Autodesk Fusion 360 part; units mm, degrees
(part 4 of 7)
  spline S44 degree 5 poles (-7.921, 8.6736) (-7.9244, 8.6773) (-7.9314, 8.6848) (-7.9421, 8.6957) (-7.957, 8.7098) (-7.9762, 8.7266) (-7.9959, 8.743) (-8.016, 8.759) (-8.0362, 8.7749) (-8.0566, 8.7907) (-8.077, 8.8063) (-8.0977, 8.8219) (-8.1185, 8.8372) (-8.1396, 8.8522) (-8.1609, 8.867) (-8.1824, 8.8816) (-8.2042, 8.896) (-8.226, 8.9102) (-8.2481, 8.9242) (-8.2702, 8.9382) (-8.2925, 8.9519) (-8.3149, 8.9656) (-8.3375, 8.9791) (-8.3602, 8.9924) (-8.3831, 9.0056) (-8.4061, 9.0186) (-8.4292, 9.0314) (-8.4524, 9.0442) (-8.4758, 9.0568) (-8.4993, 9.0692) (-8.5229, 9.0816) (-8.5466, 9.0938) (-8.5704, 9.1058) (-8.5943, 9.1178) (-8.6184, 9.1296) (-8.6426, 9.1413) (-8.6668, 9.1528) (-8.6912, 9.1642) (-8.7157, 9.1755) (-8.7402, 9.1867) (-8.7649, 9.1978) (-8.7897, 9.2087) (-8.8146, 9.2195) (-8.8395, 9.2302) (-8.8646, 9.2408) (-8.8897, 9.2512) (-8.915, 9.2616) (-8.9403, 9.2718) (-8.9658, 9.2819) (-8.9913, 9.2919) (-9.0169, 9.3018) (-9.0426, 9.3115) (-9.0684, 9.3212) (-9.0942, 9.3307) (-9.1202, 9.3401) (-9.1462, 9.3494) (-9.1723, 9.3586) (-9.1985, 9.3677) (-9.2248, 9.3767) (-9.2512, 9.3856) (-9.2776, 9.3943) (-9.3041, 9.403) (-9.3307, 9.4115) (-9.3574, 9.4199) (-9.3841, 9.4282) (-9.4109, 9.4364) (-9.4378, 9.4445) (-9.4648, 9.4525) (-9.4918, 9.4604) (-9.5189, 9.4682) (-9.5461, 9.4758) (-9.5679, 9.4819) (-9.5843, 9.4864) (-9.5953, 9.4894) (-9.6007, 9.4908) knots 0 0 0 0 0 0 0.01428571 0.02857143 0.04285714 0.05714286 0.07142857 0.08571429 0.1 0.11428571 0.12857143 0.14285714 0.15714286 0.17142857 0.18571429 0.2 0.21428571 0.22857143 0.24285714 0.25714286 0.27142857 0.28571429 0.3 0.31428571 0.32857143 0.34285714 0.35714286 0.37142857 0.38571429 0.4 0.41428571 0.42857143 0.44285714 0.45714286 0.47142857 0.48571429 0.5 0.51428571 0.52857143 0.54285714 0.55714286 0.57142857 0.58571429 0.6 0.61428571 0.62857143 0.64285714 0.65714286 0.67142857 0.68571429 0.7 0.71428571 0.72857143 0.74285714 0.75714286 0.77142857 0.78571429 0.8 0.81428571 0.82857143 0.84285714 0.85714286 0.87142857 0.88571429 0.9 0.91428571 0.92857143 0.94285714 0.95714286 0.97142857 0.98571429 1 1 1 1 1 1
  arc A90 (-9.6007, 9.4908) -> (-10.0749, 8.9858) centre (0, 0) ccw
  spline S45 degree 5 poles (-10.0749, 8.9858) (-10.0731, 8.9805) (-10.0695, 8.9698) (-10.064, 8.9537) (-10.0566, 8.9323) (-10.0472, 8.9057) (-10.0377, 8.8791) (-10.0282, 8.8526) (-10.0185, 8.8262) (-10.0087, 8.7998) (-9.9989, 8.7736) (-9.9889, 8.7474) (-9.9788, 8.7213) (-9.9686, 8.6953) (-9.9583, 8.6694) (-9.9479, 8.6436) (-9.9374, 8.6178) (-9.9268, 8.5922) (-9.9161, 8.5666) (-9.9053, 8.5411) (-9.8944, 8.5157) (-9.8833, 8.4904) (-9.8722, 8.4652) (-9.8609, 8.4401) (-9.8496, 8.415) (-9.8381, 8.3901) (-9.8266, 8.3653) (-9.8149, 8.3405) (-9.8031, 8.3159) (-9.7912, 8.2913) (-9.7792, 8.2669) (-9.767, 8.2425) (-9.7548, 8.2183) (-9.7424, 8.1941) (-9.73, 8.1701) (-9.7174, 8.1462) (-9.7047, 8.1223) (-9.6919, 8.0986) (-9.6789, 8.075) (-9.6659, 8.0515) (-9.6527, 8.0281) (-9.6394, 8.0049) (-9.626, 7.9817) (-9.6125, 7.9587) (-9.5988, 7.9358) (-9.585, 7.913) (-9.5711, 7.8904) (-9.5571, 7.8679) (-9.5429, 7.8455) (-9.5286, 7.8232) (-9.5142, 7.8011) (-9.4996, 7.7791) (-9.4849, 7.7572) (-9.47, 7.7356) (-9.455, 7.7141) (-9.4398, 7.6927) (-9.4245, 7.6714) (-9.4091, 7.6503) (-9.3936, 7.6294) (-9.3779, 7.6086) (-9.362, 7.588) (-9.3458, 7.5677) (-9.3295, 7.5476) (-9.3129, 7.5278) (-9.2961, 7.5081) (-9.2792, 7.4887) (-9.2622, 7.4694) (-9.2451, 7.4502) (-9.2278, 7.4312) (-9.2102, 7.4125) (-9.1922, 7.3944) (-9.1772, 7.3805) (-9.1657, 7.3704) (-9.1578, 7.3639) (-9.1538, 7.3607) knots -1 -1 -1 -1 -1 -1 -0.98571429 -0.97142857 -0.95714286 -0.94285714 -0.92857143 -0.91428571 -0.9 -0.88571429 -0.87142857 -0.85714286 -0.84285714 -0.82857143 -0.81428571 -0.8 -0.78571429 -0.77142857 -0.75714286 -0.74285714 -0.72857143 -0.71428571 -0.7 -0.68571429 -0.67142857 -0.65714286 -0.64285714 -0.62857143 -0.61428571 -0.6 -0.58571429 -0.57142857 -0.55714286 -0.54285714 -0.52857143 -0.51428571 -0.5 -0.48571429 -0.47142857 -0.45714286 -0.44285714 -0.42857143 -0.41428571 -0.4 -0.38571429 -0.37142857 -0.35714286 -0.34285714 -0.32857143 -0.31428571 -0.3 -0.28571429 -0.27142857 -0.25714286 -0.24285714 -0.22857143 -0.21428571 -0.2 -0.18571429 -0.17142857 -0.15714286 -0.14285714 -0.12857143 -0.11428571 -0.1 -0.08571429 -0.07142857 -0.05714286 -0.04285714 -0.02857143 -0.01428571 0 0 0 0 0 0
  line L45 (-9.1538, 7.3607) -> (-9.0704, 7.2937)
  arc A91 (-9.0198, 6.878) -> (-9.0704, 7.2937) centre (-9.2584, 7.0599) ccw
  arc A92 (-9.0198, 6.878) -> (-9.3286, 6.453) centre (0, 0) ccw
  arc A93 (-9.7396, 6.3726) -> (-9.3286, 6.453) centre (-9.5753, 6.6236) ccw
  line L46 (-9.7396, 6.3726) -> (-9.8291, 6.4312)
  spline S46 degree 5 poles (-9.8291, 6.4312) (-9.8334, 6.434) (-9.842, 6.4395) (-9.8551, 6.4474) (-9.873, 6.4573) (-9.8958, 6.4689) (-9.919, 6.4798) (-9.9424, 6.4904) (-9.966, 6.5007) (-9.9896, 6.5109) (-10.0133, 6.521) (-10.0372, 6.5309) (-10.0612, 6.5405) (-10.0853, 6.5499) (-10.1096, 6.5589) (-10.1341, 6.5677) (-10.1587, 6.5762) (-10.1835, 6.5845) (-10.2083, 6.5927) (-10.2332, 6.6006) (-10.2582, 6.6084) (-10.2834, 6.6161) (-10.3086, 6.6235) (-10.3339, 6.6308) (-10.3593, 6.6379) (-10.3848, 6.6447) (-10.4104, 6.6515) (-10.4361, 6.658) (-10.4618, 6.6644) (-10.4877, 6.6706) (-10.5136, 6.6767) (-10.5396, 6.6826) (-10.5657, 6.6884) (-10.5918, 6.694) (-10.6181, 6.6995) (-10.6444, 6.7048) (-10.6707, 6.7099) (-10.6972, 6.7149) (-10.7237, 6.7198) (-10.7503, 6.7245) (-10.7769, 6.7291) (-10.8037, 6.7335) (-10.8304, 6.7378) (-10.8573, 6.7419) (-10.8842, 6.7459) (-10.9111, 6.7498) (-10.9382, 6.7535) (-10.9653, 6.7571) (-10.9924, 6.7606) (-11.0196, 6.7639) (-11.0469, 6.7671) (-11.0742, 6.7702) (-11.1015, 6.7731) (-11.129, 6.7759) (-11.1564, 6.7786) (-11.184, 6.7811) (-11.2116, 6.7836) (-11.2392, 6.7858) (-11.2669, 6.788) (-11.2946, 6.79) (-11.3224, 6.7919) (-11.3502, 6.7937) (-11.3781, 6.7954) (-11.406, 6.7969) (-11.434, 6.7983) (-11.462, 6.7996) (-11.4901, 6.8007) (-11.5182, 6.8018) (-11.5463, 6.8027) (-11.5745, 6.8035) (-11.6028, 6.8041) (-11.6254, 6.8046) (-11.6424, 6.8048) (-11.6537, 6.805) (-11.6594, 6.8051) knots 0 0 0 0 0 0 0.01428571 0.02857143 0.04285714 0.05714286 0.07142857 0.08571429 0.1 0.11428571 0.12857143 0.14285714 0.15714286 0.17142857 0.18571429 0.2 0.21428571 0.22857143 0.24285714 0.25714286 0.27142857 0.28571429 0.3 0.31428571 0.32857143 0.34285714 0.35714286 0.37142857 0.38571429 0.4 0.41428571 0.42857143 0.44285714 0.45714286 0.47142857 0.48571429 0.5 0.51428571 0.52857143 0.54285714 0.55714286 0.57142857 0.58571429 0.6 0.61428571 0.62857143 0.64285714 0.65714286 0.67142857 0.68571429 0.7 0.71428571 0.72857143 0.74285714 0.75714286 0.77142857 0.78571429 0.8 0.81428571 0.82857143 0.84285714 0.85714286 0.87142857 0.88571429 0.9 0.91428571 0.92857143 0.94285714 0.95714286 0.97142857 0.98571429 1 1 1 1 1 1
  arc A94 (-11.6594, 6.8051) -> (-11.9931, 6.198) centre (0, 0) ccw
  spline S47 degree 5 poles (-11.9931, 6.198) (-11.99, 6.1933) (-11.9838, 6.1838) (-11.9745, 6.1696) (-11.962, 6.1507) (-11.9463, 6.1272) (-11.9305, 6.1038) (-11.9147, 6.0806) (-11.8987, 6.0574) (-11.8827, 6.0343) (-11.8666, 6.0113) (-11.8505, 5.9885) (-11.8342, 5.9657) (-11.8179, 5.9431) (-11.8015, 5.9205) (-11.785, 5.8981) (-11.7684, 5.8757) (-11.7517, 5.8535) (-11.735, 5.8314) (-11.7182, 5.8094) (-11.7013, 5.7875) (-11.6843, 5.7658) (-11.6672, 5.7441) (-11.6501, 5.7226) (-11.6329, 5.7012) (-11.6156, 5.6799) (-11.5982, 5.6587) (-11.5807, 5.6376) (-11.5632, 5.6167) (-11.5455, 5.5959) (-11.5278, 5.5752) (-11.51, 5.5546) (-11.4921, 5.5342) (-11.4742, 5.5138) (-11.4561, 5.4937) (-11.438, 5.4736) (-11.4197, 5.4537) (-11.4014, 5.4339) (-11.383, 5.4143) (-11.3646, 5.3948) (-11.346, 5.3754) (-11.3273, 5.3562) (-11.3086, 5.3371) (-11.2897, 5.3182) (-11.2708, 5.2994) (-11.2518, 5.2807) (-11.2327, 5.2623) (-11.2135, 5.2439) (-11.1942, 5.2258) (-11.1748, 5.2077) (-11.1553, 5.1899) (-11.1357, 5.1722) (-11.116, 5.1547) (-11.0962, 5.1375) (-11.0763, 5.1203) (-11.0563, 5.1034) (-11.0362, 5.0866) (-11.0161, 5.07) (-10.9958, 5.0536) (-10.9754, 5.0374) (-10.9549, 5.0214) (-10.9342, 5.0057) (-10.9134, 4.9903) (-10.8924, 4.9752) (-10.8713, 4.9604) (-10.85, 4.9458) (-10.8288, 4.9313) (-10.8074, 4.917) (-10.7859, 4.9028) (-10.7643, 4.8891) (-10.7423, 4.8761) (-10.7244, 4.8663) (-10.7107, 4.8595) (-10.7014, 4.8551) (-10.6968, 4.853) knots -1 -1 -1 -1 -1 -1 -0.98571429 -0.97142857 -0.95714286 -0.94285714 -0.92857143 -0.91428571 -0.9 -0.88571429 -0.87142857 -0.85714286 -0.84285714 -0.82857143 -0.81428571 -0.8 -0.78571429 -0.77142857 -0.75714286 -0.74285714 -0.72857143 -0.71428571 -0.7 -0.68571429 -0.67142857 -0.65714286 -0.64285714 -0.62857143 -0.61428571 -0.6 -0.58571429 -0.57142857 -0.55714286 -0.54285714 -0.52857143 -0.51428571 -0.5 -0.48571429 -0.47142857 -0.45714286 -0.44285714 -0.42857143 -0.41428571 -0.4 -0.38571429 -0.37142857 -0.35714286 -0.34285714 -0.32857143 -0.31428571 -0.3 -0.28571429 -0.27142857 -0.25714286 -0.24285714 -0.22857143 -0.21428571 -0.2 -0.18571429 -0.17142857 -0.15714286 -0.14285714 -0.12857143 -0.11428571 -0.1 -0.08571429 -0.07142857 -0.05714286 -0.04285714 -0.02857143 -0.01428571 0 0 0 0 0 0
  line L47 (-10.6968, 4.853) -> (-10.5993, 4.8088)
  arc A95 (-10.4469, 4.4187) -> (-10.5993, 4.8088) centre (-10.7232, 4.5356) ccw
  arc A96 (-10.4469, 4.4187) -> (-10.6403, 3.9303) centre (0, 0) ccw
  arc A97 (-11.0184, 3.7503) -> (-10.6403, 3.9303) centre (-10.9217, 4.0343) ccw
  line L48 (-11.0184, 3.7503) -> (-11.1197, 3.7847)
  spline S48 degree 5 poles (-11.1197, 3.7847) (-11.1245, 3.7864) (-11.1343, 3.7896) (-11.1489, 3.794) (-11.1687, 3.7991) (-11.1937, 3.8046) (-11.2188, 3.8095) (-11.2441, 3.8139) (-11.2695, 3.818) (-11.295, 3.8221) (-11.3205, 3.8259) (-11.346, 3.8296) (-11.3716, 3.8329) (-11.3974, 3.836) (-11.4232, 3.8387) (-11.4491, 3.8411) (-11.475, 3.8432) (-11.501, 3.8451) (-11.5271, 3.8468) (-11.5532, 3.8484) (-11.5794, 3.8497) (-11.6056, 3.8508) (-11.6319, 3.8518) (-11.6582, 3.8525) (-11.6846, 3.8531) (-11.711, 3.8534) (-11.7375, 3.8535) (-11.764, 3.8535) (-11.7905, 3.8533) (-11.8171, 3.8529) (-11.8437, 3.8523) (-11.8704, 3.8516) (-11.8971, 3.8507) (-11.9238, 3.8496) (-11.9506, 3.8484) (-11.9774, 3.847) (-12.0042, 3.8454) (-12.0311, 3.8437) (-12.0579, 3.8418) (-12.0849, 3.8397) (-12.1118, 3.8375) (-12.1388, 3.8352) (-12.1658, 3.8327) (-12.1928, 3.83) (-12.2199, 3.8272) (-12.247, 3.8243) (-12.2741, 3.8212) (-12.3012, 3.8179) (-12.3283, 3.8145) (-12.3555, 3.811) (-12.3827, 3.8073) (-12.4099, 3.8035) (-12.4372, 3.7995) (-12.4644, 3.7954) (-12.4917, 3.7911) (-12.519, 3.7868) (-12.5463, 3.7822) (-12.5737, 3.7776) (-12.601, 3.7728) (-12.6284, 3.7678) (-12.6558, 3.7628) (-12.6832, 3.7576) (-12.7106, 3.7522) (-12.738, 3.7468) (-12.7654, 3.7412) (-12.7929, 3.7355) (-12.8204, 3.7296) (-12.8478, 3.7236) (-12.8753, 3.7175) (-12.9028, 3.7112) (-12.9304, 3.7049) (-12.9524, 3.6997) (-12.9689, 3.6957) (-12.9799, 3.693) (-12.9854, 3.6917) knots 0 0 0 0 0 0 0.01428571 0.02857143 0.04285714 0.05714286 0.07142857 0.08571429 0.1 0.11428571 0.12857143 0.14285714 0.15714286 0.17142857 0.18571429 0.2 0.21428571 0.22857143 0.24285714 0.25714286 0.27142857 0.28571429 0.3 0.31428571 0.32857143 0.34285714 0.35714286 0.37142857 0.38571429 0.4 0.41428571 0.42857143 0.44285714 0.45714286 0.47142857 0.48571429 0.5 0.51428571 0.52857143 0.54285714 0.55714286 0.57142857 0.58571429 0.6 0.61428571 0.62857143 0.64285714 0.65714286 0.67142857 0.68571429 0.7 0.71428571 0.72857143 0.74285714 0.75714286 0.77142857 0.78571429 0.8 0.81428571 0.82857143 0.84285714 0.85714286 0.87142857 0.88571429 0.9 0.91428571 0.92857143 0.94285714 0.95714286 0.97142857 0.98571429 1 1 1 1 1 1
  arc A98 (-12.9854, 3.6917) -> (-13.1577, 3.0207) centre (0, 0) ccw
  spline S49 degree 5 poles (-13.1577, 3.0207) (-13.1535, 3.0169) (-13.1452, 3.0092) (-13.1326, 2.9978) (-13.1158, 2.9827) (-13.0948, 2.9638) (-13.0737, 2.9451) (-13.0525, 2.9265) (-13.0313, 2.908) (-13.0101, 2.8896) (-12.9888, 2.8714) (-12.9674, 2.8532) (-12.946, 2.8352) (-12.9246, 2.8174) (-12.9031, 2.7996) (-12.8815, 2.782) (-12.8599, 2.7645) (-12.8382, 2.7471) (-12.8165, 2.7298) (-12.7948, 2.7127) (-12.773, 2.6957) (-12.7511, 2.6789) (-12.7292, 2.6621) (-12.7072, 2.6455) (-12.6852, 2.6291) (-12.6632, 2.6127) (-12.6411, 2.5965) (-12.6189, 2.5805) (-12.5967, 2.5646) (-12.5744, 2.5488) (-12.5521, 2.5332) (-12.5298, 2.5177) (-12.5074, 2.5023) (-12.4849, 2.4871) (-12.4624, 2.4721) (-12.4399, 2.4571) (-12.4172, 2.4424) (-12.3946, 2.4278) (-12.3719, 2.4133) (-12.3491, 2.399) (-12.3263, 2.3849) (-12.3035, 2.3709) (-12.2806, 2.3571) (-12.2576, 2.3434) (-12.2346, 2.33) (-12.2115, 2.3166) (-12.1884, 2.3035) (-12.1653, 2.2905) (-12.1421, 2.2777) (-12.1188, 2.2651) (-12.0955, 2.2526) (-12.0722, 2.2404) (-12.0487, 2.2284) (-12.0253, 2.2165) (-12.0017, 2.2049) (-11.9781, 2.1935) (-11.9545, 2.1822) (-11.9308, 2.1712) (-11.9071, 2.1603) (-11.8833, 2.1496) (-11.8595, 2.1393) (-11.8356, 2.1292) (-11.8116, 2.1195) (-11.7875, 2.1101) (-11.7633, 2.101) (-11.7391, 2.0921) (-11.7149, 2.0834) (-11.6907, 2.0748) (-11.6664, 2.0665) (-11.642, 2.0586) (-11.6174, 2.0514) (-11.5976, 2.0464) (-11.5827, 2.0432) (-11.5726, 2.0413) (-11.5676, 2.0404) knots -1 -1 -1 -1 -1 -1 -0.98571429 -0.97142857 -0.95714286 -0.94285714 -0.92857143 -0.91428571 -0.9 -0.88571429 -0.87142857 -0.85714286 -0.84285714 -0.82857143 -0.81428571 -0.8 -0.78571429 -0.77142857 -0.75714286 -0.74285714 -0.72857143 -0.71428571 -0.7 -0.68571429 -0.67142857 -0.65714286 -0.64285714 -0.62857143 -0.61428571 -0.6 -0.58571429 -0.57142857 -0.55714286 -0.54285714 -0.52857143 -0.51428571 -0.5 -0.48571429 -0.47142857 -0.45714286 -0.44285714 -0.42857143 -0.41428571 -0.4 -0.38571429 -0.37142857 -0.35714286 -0.34285714 -0.32857143 -0.31428571 -0.3 -0.28571429 -0.27142857 -0.25714286 -0.24285714 -0.22857143 -0.21428571 -0.2 -0.18571429 -0.17142857 -0.15714286 -0.14285714 -0.12857143 -0.11428571 -0.1 -0.08571429 -0.07142857 -0.05714286 -0.04285714 -0.02857143 -0.01428571 0 0 0 0 0 0
  line L49 (-11.5676, 2.0404) -> (-11.4622, 2.0218)
  arc A99 (-11.2176, 1.6819) -> (-11.4622, 2.0218) centre (-11.5143, 1.7263) ccw
  circle A100 centre (0, 0) radius 2.6
  circle A101 centre (7.5749, -4.8601) radius 1.1
  circle A102 centre (8.9849, 0.5205) radius 1.1
  circle A103 centre (6.963, 5.7023) radius 1.1
  circle A104 centre (2.2815, 8.706) radius 1.1
  circle A105 centre (-3.2715, 8.3843) radius 1.1
  circle A106 centre (-7.5749, 4.8601) radius 1.1
  circle A107 centre (-8.9849, -0.5205) radius 1.1
  circle A108 centre (-6.963, -5.7023) radius 1.1
  circle A109 centre (-2.2815, -8.706) radius 1.1
  circle A110 centre (3.2715, -8.3843) radius 1.1
  dimension "d31" = 2.2
  dimension "d32" = 9
  dimension "d34" = 360
  dimension "d36" = 4.6816
  measures "d31" diameter of A101
  measures "d32" distance of A0.centre A101.centre
  measures "d36" horizontal distance of A103.centre A104.centre
extrude "Extrude8" cut sketch "gauri flaps" against normal up to surface (5 mm away) contours A101 | A102 | A103 | A104 | A105 | A106 | A107 | A108 | A109 | A110
sketch "Base Circle (2)" plane through (0, 0, 0) normal (0, 0, 1) x (1, 0, 0)
  circle A0 centre (0, 0) radius 8.843
  circle A1 centre (0, 0) radius 2.6
extrude "Extrude4" [suppressed]
sketch "Gear Tooth (2)" plane through (0, 0, 0) normal (0, 0, 1) x (1, 0, 0)
  spline S0 degree 5 poles (9.357, -0.8651) (9.3617, -0.8655) (9.371, -0.8663) (9.385, -0.867) (9.4037, -0.8673) (9.4271, -0.8667) (9.4506, -0.8654) (9.474, -0.8636) (9.4975, -0.8616) (9.5211, -0.8595) (9.5446, -0.8572) (9.5681, -0.8546) (9.5917, -0.8518) (9.6152, -0.8487) (9.6388, -0.8452) (9.6624, -0.8414) (9.686, -0.8373) (9.7095, -0.833) (9.7331, -0.8285) (9.7567, -0.8238) (9.7803, -0.8189) (9.8039, -0.8138) (9.8275, -0.8085) (9.8511, -0.803) (9.8747, -0.7973) (9.8983, -0.7914) (9.9219, -0.7853) (9.9454, -0.779) (9.969, -0.7725) (9.9926, -0.7658) (10.0162, -0.759) (10.0397, -0.752) (10.0633, -0.7448) (10.0868, -0.7375) (10.1104, -0.73) (10.1339, -0.7223) (10.1574, -0.7144) (10.181, -0.7064) (10.2045, -0.6982) (10.228, -0.6899) (10.2515, -0.6814) (10.2749, -0.6728) (10.2984, -0.664) (10.3218, -0.655) (10.3453, -0.6459) (10.3687, -0.6367) (10.3921, -0.6273) (10.4155, -0.6177) (10.4389, -0.608) (10.4623, -0.5982) (10.4857, -0.5882) (10.509, -0.578) (10.5323, -0.5678) (10.5556, -0.5573) (10.5789, -0.5468) (10.6022, -0.5361) (10.6255, -0.5252) (10.6487, -0.5143) (10.6719, -0.5032) (10.6951, -0.4919) (10.7183, -0.4805) (10.7415, -0.469) (10.7646, -0.4574) (10.7878, -0.4456) (10.8109, -0.4337) (10.834, -0.4216) (10.857, -0.4094) (10.8801, -0.3971) (10.9031, -0.3847) (10.9261, -0.3721) (10.9491, -0.3594) (10.9674, -0.3492) (10.9812, -0.3414) (10.9904, -0.3362) (10.9949, -0.3336) knots 0 0 0 0 0 0 0.01428571 0.02857143 0.04285714 0.05714286 0.07142857 0.08571429 0.1 0.11428571 0.12857143 0.14285714 0.15714286 0.17142857 0.18571429 0.2 0.21428571 0.22857143 0.24285714 0.25714286 0.27142857 0.28571429 0.3 0.31428571 0.32857143 0.34285714 0.35714286 0.37142857 0.38571429 0.4 0.41428571 0.42857143 0.44285714 0.45714286 0.47142857 0.48571429 0.5 0.51428571 0.52857143 0.54285714 0.55714286 0.57142857 0.58571429 0.6 0.61428571 0.62857143 0.64285714 0.65714286 0.67142857 0.68571429 0.7 0.71428571 0.72857143 0.74285714 0.75714286 0.77142857 0.78571429 0.8 0.81428571 0.82857143 0.84285714 0.85714286 0.87142857 0.88571429 0.9 0.91428571 0.92857143 0.94285714 0.95714286 0.97142857 0.98571429 1 1 1 1 1 1
  spline S1 degree 5 poles (9.357, 0.8651) (9.3617, 0.8655) (9.371, 0.8663) (9.385, 0.867) (9.4037, 0.8673) (9.4271, 0.8667) (9.4506, 0.8654) (9.474, 0.8636) (9.4975, 0.8616) (9.5211, 0.8595) (9.5446, 0.8572) (9.5681, 0.8546) (9.5917, 0.8518) (9.6152, 0.8487) (9.6388, 0.8452) (9.6624, 0.8414) (9.686, 0.8373) (9.7095, 0.833) (9.7331, 0.8285) (9.7567, 0.8238) (9.7803, 0.8189) (9.8039, 0.8138) (9.8275, 0.8085) (9.8511, 0.803) (9.8747, 0.7973) (9.8983, 0.7914) (9.9219, 0.7853) (9.9454, 0.779) (9.969, 0.7725) (9.9926, 0.7658) (10.0162, 0.759) (10.0397, 0.752) (10.0633, 0.7448) (10.0868, 0.7375) (10.1104, 0.73) (10.1339, 0.7223) (10.1574, 0.7144) (10.181, 0.7064) (10.2045, 0.6982) (10.228, 0.6899) (10.2515, 0.6814) (10.2749, 0.6728) (10.2984, 0.664) (10.3218, 0.655) (10.3453, 0.6459) (10.3687, 0.6367) (10.3921, 0.6273) (10.4155, 0.6177) (10.4389, 0.608) (10.4623, 0.5982) (10.4857, 0.5882) (10.509, 0.578) (10.5323, 0.5678) (10.5556, 0.5573) (10.5789, 0.5468) (10.6022, 0.5361) (10.6255, 0.5252) (10.6487, 0.5143) (10.6719, 0.5032) (10.6951, 0.4919) (10.7183, 0.4805) (10.7415, 0.469) (10.7646, 0.4574) (10.7878, 0.4456) (10.8109, 0.4337) (10.834, 0.4216) (10.857, 0.4094) (10.8801, 0.3971) (10.9031, 0.3847) (10.9261, 0.3721) (10.9491, 0.3594) (10.9674, 0.3492) (10.9812, 0.3414) (10.9904, 0.3362) (10.9949, 0.3336) knots 0 0 0 0 0 0 0.01428571 0.02857143 0.04285714 0.05714286 0.07142857 0.08571429 0.1 0.11428571 0.12857143 0.14285714 0.15714286 0.17142857 0.18571429 0.2 0.21428571 0.22857143 0.24285714 0.25714286 0.27142857 0.28571429 0.3 0.31428571 0.32857143 0.34285714 0.35714286 0.37142857 0.38571429 0.4 0.41428571 0.42857143 0.44285714 0.45714286 0.47142857 0.48571429 0.5 0.51428571 0.52857143 0.54285714 0.55714286 0.57142857 0.58571429 0.6 0.61428571 0.62857143 0.64285714 0.65714286 0.67142857 0.68571429 0.7 0.71428571 0.72857143 0.74285714 0.75714286 0.77142857 0.78571429 0.8 0.81428571 0.82857143 0.84285714 0.85714286 0.87142857 0.88571429 0.9 0.91428571 0.92857143 0.94285714 0.95714286 0.97142857 0.98571429 1 1 1 1 1 1
  arc A0 (10.9949, -0.3336) -> (10.9949, 0.3336) centre (0, 0) ccw
  line L0 (8.7955, -0.8132) -> (9.357, -0.8651)
  line L1 (8.7955, 0.8132) -> (9.357, 0.8651)
  line L2 (8.7955, -0.8132) -> (8.7955, 0.8132)
  point P0 (9.4721, -0.8637)
  point P1 (9.5881, -0.8522)
  point P2 (9.7047, -0.8338)
  point P3 (9.8216, -0.8098)
  point P4 (9.9388, -0.7807)
  point P5 (10.0563, -0.7469)
  point P6 (10.1738, -0.7088)
  point P7 (10.2914, -0.6666)
  point P8 (10.409, -0.6203)
  point P9 (10.5265, -0.5703)
  point P10 (10.644, -0.5165)
  point P11 (10.7612, -0.4591)
  point P12 (10.8782, -0.3981)
  point P13 (9.4721, 0.8637)
  point P14 (9.5881, 0.8522)
  point P15 (9.7047, 0.8338)
  point P16 (9.8216, 0.8098)
  point P17 (9.9388, 0.7807)
  point P18 (10.0563, 0.7469)
  point P19 (10.1738, 0.7088)
  point P20 (10.2914, 0.6666)
  point P21 (10.409, 0.6203)
  point P22 (10.5265, 0.5703)
  point P23 (10.644, 0.5165)
  point P24 (10.7612, 0.4591)
  point P25 (10.8782, 0.3981)
extrude "Extrude5" [suppressed]
fillet "Fillet2" [suppressed]
pattern_circular "C-Pattern2" [suppressed]
sketch "Diametrial Pitch Circle (2)" plane through (0, 0, 0) normal (0, 0, 1) x (1, 0, 0)
  circle A0 centre (0, 0) radius 10 construction
sketch "Sketch7" plane through (0, 0, 5) normal (0, 0, 1) x (-1, 0, 0)
  arc A0 (-8.6853, 1.6627) -> (-8.774, 1.1026) centre (0, 0) ccw
  arc A1 (-9.0993, 0.8413) -> (-8.774, 1.1026) centre (-9.0716, 1.14) ccw
  line L0 (-9.0993, 0.8413) -> (-9.357, 0.8651)
  spline S0 degree 5 poles (-9.357, 0.8651) (-9.3617, 0.8655) (-9.371, 0.8663) (-9.385, 0.867) (-9.4037, 0.8673) (-9.4271, 0.8667) (-9.4506, 0.8654) (-9.474, 0.8636) (-9.4975, 0.8616) (-9.5211, 0.8595) (-9.5446, 0.8572) (-9.5681, 0.8546) (-9.5917, 0.8518) (-9.6152, 0.8487) (-9.6388, 0.8452) (-9.6624, 0.8414) (-9.686, 0.8373) (-9.7095, 0.833) (-9.7331, 0.8285) (-9.7567, 0.8238) (-9.7803, 0.8189) (-9.8039, 0.8138) (-9.8275, 0.8085) (-9.8511, 0.803) (-9.8747, 0.7973) (-9.8983, 0.7914) (-9.9219, 0.7853) (-9.9454, 0.779) (-9.969, 0.7725) (-9.9926, 0.7658) (-10.0162, 0.759) (-10.0397, 0.752) (-10.0633, 0.7448) (-10.0868, 0.7375) (-10.1104, 0.73) (-10.1339, 0.7223) (-10.1574, 0.7144) (-10.181, 0.7064) (-10.2045, 0.6982) (-10.228, 0.6899) (-10.2515, 0.6814) (-10.2749, 0.6728) (-10.2984, 0.664) (-10.3218, 0.655) (-10.3453, 0.6459) (-10.3687, 0.6367) (-10.3921, 0.6273) (-10.4155, 0.6177) (-10.4389, 0.608) (-10.4623, 0.5982) (-10.4857, 0.5882) (-10.509, 0.578) (-10.5323, 0.5678) (-10.5556, 0.5573) (-10.5789, 0.5468) (-10.6022, 0.5361) (-10.6255, 0.5252) (-10.6487, 0.5143) (-10.6719, 0.5032) (-10.6951, 0.4919) (-10.7183, 0.4805) (-10.7415, 0.469) (-10.7646, 0.4574) (-10.7878, 0.4456) (-10.8109, 0.4337) (-10.834, 0.4216) (-10.857, 0.4094) (-10.8801, 0.3971) (-10.9031, 0.3847) (-10.9261, 0.3721) (-10.9491, 0.3594) (-10.9674, 0.3492) (-10.9812, 0.3414) (-10.9904, 0.3362) (-10.9949, 0.3336) knots 0 0 0 0 0 0 0.01428571 0.02857143 0.04285714 0.05714286 0.07142857 0.08571429 0.1 0.11428571 0.12857143 0.14285714 0.15714286 0.17142857 0.18571429 0.2 0.21428571 0.22857143 0.24285714 0.25714286 0.27142857 0.28571429 0.3 0.31428571 0.32857143 0.34285714 0.35714286 0.37142857 0.38571429 0.4 0.41428571 0.42857143 0.44285714 0.45714286 0.47142857 0.48571429 0.5 0.51428571 0.52857143 0.54285714 0.55714286 0.57142857 0.58571429 0.6 0.61428571 0.62857143 0.64285714 0.65714286 0.67142857 0.68571429 0.7 0.71428571 0.72857143 0.74285714 0.75714286 0.77142857 0.78571429 0.8 0.81428571 0.82857143 0.84285714 0.85714286 0.87142857 0.88571429 0.9 0.91428571 0.92857143 0.94285714 0.95714286 0.97142857 0.98571429 1 1 1 1 1 1
  arc A2 (-10.9949, 0.3336) -> (-10.9949, -0.3336) centre (0, 0) ccw
  spline S1 degree 5 poles (-10.9949, -0.3336) (-10.9904, -0.3362) (-10.9812, -0.3414) (-10.9674, -0.3492) (-10.9491, -0.3594) (-10.9261, -0.3721) (-10.9031, -0.3847) (-10.8801, -0.3971) (-10.857, -0.4094) (-10.834, -0.4216) (-10.8109, -0.4337) (-10.7878, -0.4456) (-10.7646, -0.4574) (-10.7415, -0.469) (-10.7183, -0.4805) (-10.6951, -0.4919) (-10.6719, -0.5032) (-10.6487, -0.5143) (-10.6255, -0.5252) (-10.6022, -0.5361) (-10.5789, -0.5468) (-10.5556, -0.5573) (-10.5323, -0.5678) (-10.509, -0.578) (-10.4857, -0.5882) (-10.4623, -0.5982) (-10.4389, -0.608) (-10.4155, -0.6177) (-10.3921, -0.6273) (-10.3687, -0.6367) (-10.3453, -0.6459) (-10.3218, -0.655) (-10.2984, -0.664) (-10.2749, -0.6728) (-10.2515, -0.6814) (-10.228, -0.6899) (-10.2045, -0.6982) (-10.181, -0.7064) (-10.1574, -0.7144) (-10.1339, -0.7223) (-10.1104, -0.73) (-10.0868, -0.7375) (-10.0633, -0.7448) (-10.0397, -0.752) (-10.0162, -0.759) (-9.9926, -0.7658) (-9.969, -0.7725) (-9.9454, -0.779) (-9.9219, -0.7853) (-9.8983, -0.7914) (-9.8747, -0.7973) (-9.8511, -0.803) (-9.8275, -0.8085) (-9.8039, -0.8138) (-9.7803, -0.8189) (-9.7567, -0.8238) (-9.7331, -0.8285) (-9.7095, -0.833) (-9.686, -0.8373) (-9.6624, -0.8414) (-9.6388, -0.8452) (-9.6152, -0.8487) (-9.5917, -0.8518) (-9.5681, -0.8546) (-9.5446, -0.8572) (-9.5211, -0.8595) (-9.4975, -0.8616) (-9.474, -0.8636) (-9.4506, -0.8654) (-9.4271, -0.8667) (-9.4037, -0.8673) (-9.385, -0.867) (-9.371, -0.8663) (-9.3617, -0.8655) (-9.357, -0.8651) knots -1 -1 -1 -1 -1 -1 -0.98571429 -0.97142857 -0.95714286 -0.94285714 -0.92857143 -0.91428571 -0.9 -0.88571429 -0.87142857 -0.85714286 -0.84285714 -0.82857143 -0.81428571 -0.8 -0.78571429 -0.77142857 -0.75714286 -0.74285714 -0.72857143 -0.71428571 -0.7 -0.68571429 -0.67142857 -0.65714286 -0.64285714 -0.62857143 -0.61428571 -0.6 -0.58571429 -0.57142857 -0.55714286 -0.54285714 -0.52857143 -0.51428571 -0.5 -0.48571429 -0.47142857 -0.45714286 -0.44285714 -0.42857143 -0.41428571 -0.4 -0.38571429 -0.37142857 -0.35714286 -0.34285714 -0.32857143 -0.31428571 -0.3 -0.28571429 -0.27142857 -0.25714286 -0.24285714 -0.22857143 -0.21428571 -0.2 -0.18571429 -0.17142857 -0.15714286 -0.14285714 -0.12857143 -0.11428571 -0.1 -0.08571429 -0.07142857 -0.05714286 -0.04285714 -0.02857143 -0.01428571 0 0 0 0 0 0
  line L1 (-9.357, -0.8651) -> (-9.0993, -0.8413)
  arc A3 (-8.774, -1.1026) -> (-9.0993, -0.8413) centre (-9.0716, -1.14) ccw
  arc A4 (-8.774, -1.1026) -> (-8.6853, -1.6627) centre (0, 0) ccw
  arc A5 (-8.9139, -2.0117) -> (-8.6853, -1.6627) centre (-8.9799, -1.7191) ccw
  line L2 (-8.9139, -2.0117) -> (-9.1664, -2.0687)
  spline S2 degree 5 poles (-9.1664, -2.0687) (-9.171, -2.0697) (-9.1801, -2.0719) (-9.1936, -2.0755) (-9.2115, -2.0811) (-9.2335, -2.0889) (-9.2554, -2.0974) (-9.2772, -2.1063) (-9.299, -2.1154) (-9.3207, -2.1248) (-9.3423, -2.1342) (-9.3639, -2.1439) (-9.3855, -2.1539) (-9.4069, -2.1641) (-9.4282, -2.1747) (-9.4495, -2.1856) (-9.4706, -2.1968) (-9.4917, -2.2082) (-9.5128, -2.2198) (-9.5338, -2.2315) (-9.5547, -2.2435) (-9.5755, -2.2556) (-9.5964, -2.2679) (-9.6171, -2.2805) (-9.6378, -2.2932) (-9.6584, -2.3061) (-9.6789, -2.3192) (-9.6994, -2.3325) (-9.7198, -2.3459) (-9.7402, -2.3595) (-9.7605, -2.3733) (-9.7807, -2.3873) (-9.8009, -2.4014) (-9.821, -2.4156) (-9.8411, -2.43) (-9.8611, -2.4446) (-9.8811, -2.4594) (-9.901, -2.4743) (-9.9208, -2.4893) (-9.9406, -2.5045) (-9.9603, -2.5198) (-9.9799, -2.5353) (-9.9995, -2.5509) (-10.0191, -2.5667) (-10.0386, -2.5826) (-10.058, -2.5986) (-10.0773, -2.6148) (-10.0966, -2.6311) (-10.1159, -2.6476) (-10.1351, -2.6642) (-10.1542, -2.6809) (-10.1733, -2.6977) (-10.1923, -2.7147) (-10.2112, -2.7318) (-10.2301, -2.7491) (-10.249, -2.7664) (-10.2677, -2.7839) (-10.2864, -2.8015) (-10.3051, -2.8193) (-10.3237, -2.8371) (-10.3422, -2.8551) (-10.3607, -2.8732) (-10.3791, -2.8915) (-10.3975, -2.9098) (-10.4158, -2.9283) (-10.434, -2.9469) (-10.4522, -2.9656) (-10.4703, -2.9844) (-10.4883, -3.0034) (-10.5063, -3.0224) (-10.5242, -3.0416) (-10.5385, -3.057) (-10.5492, -3.0687) (-10.5564, -3.0764) (-10.5599, -3.0803) knots 0 0 0 0 0 0 0.01428571 0.02857143 0.04285714 0.05714286 0.07142857 0.08571429 0.1 0.11428571 0.12857143 0.14285714 0.15714286 0.17142857 0.18571429 0.2 0.21428571 0.22857143 0.24285714 0.25714286 0.27142857 0.28571429 0.3 0.31428571 0.32857143 0.34285714 0.35714286 0.37142857 0.38571429 0.4 0.41428571 0.42857143 0.44285714 0.45714286 0.47142857 0.48571429 0.5 0.51428571 0.52857143 0.54285714 0.55714286 0.57142857 0.58571429 0.6 0.61428571 0.62857143 0.64285714 0.65714286 0.67142857 0.68571429 0.7 0.71428571 0.72857143 0.74285714 0.75714286 0.77142857 0.78571429 0.8 0.81428571 0.82857143 0.84285714 0.85714286 0.87142857 0.88571429 0.9 0.91428571 0.92857143 0.94285714 0.95714286 0.97142857 0.98571429 1 1 1 1 1 1
  arc A6 (-10.5599, -3.0803) -> (-10.3537, -3.7149) centre (0, 0) ccw
  spline S3 degree 5 poles (-10.3537, -3.7149) (-10.3485, -3.716) (-10.3382, -3.7181) (-10.3227, -3.7212) (-10.3021, -3.7253) (-10.2763, -3.7303) (-10.2506, -3.7351) (-10.2248, -3.7398) (-10.1991, -3.7444) (-10.1734, -3.7489) (-10.1477, -3.7532) (-10.1221, -3.7574) (-10.0964, -3.7614) (-10.0708, -3.7654) (-10.0452, -3.7692) (-10.0197, -3.7728) (-9.9941, -3.7763) (-9.9686, -3.7797) (-9.9431, -3.783) (-9.9176, -3.7861) (-9.8922, -3.7891) (-9.8668, -3.7919) (-9.8414, -3.7946) (-9.816, -3.7972) (-9.7907, -3.7996) (-9.7654, -3.8019) (-9.7401, -3.804) (-9.7149, -3.806) (-9.6897, -3.8079) (-9.6645, -3.8096) (-9.6394, -3.8112) (-9.6142, -3.8126) (-9.5892, -3.8139) (-9.5641, -3.815) (-9.5391, -3.8159) (-9.5142, -3.8168) (-9.4893, -3.8174) (-9.4644, -3.8179) (-9.4395, -3.8183) (-9.4147, -3.8185) (-9.39, -3.8185) (-9.3653, -3.8184) (-9.3406, -3.8181) (-9.316, -3.8176) (-9.2914, -3.817) (-9.2669, -3.8162) (-9.2424, -3.8153) (-9.218, -3.8141) (-9.1936, -3.8128) (-9.1693, -3.8114) (-9.145, -3.8097) (-9.1208, -3.8079) (-9.0967, -3.8058) (-9.0726, -3.8035) (-9.0486, -3.8011) (-9.0246, -3.7984) (-9.0007, -3.7956) (-8.9769, -3.7926) (-8.9532, -3.7894) (-8.9295, -3.786) (-8.9059, -3.7824) (-8.8824, -3.7784) (-8.859, -3.7741) (-8.8357, -3.7695) (-8.8126, -3.7647) (-8.7895, -3.7596) (-8.7664, -3.7544) (-8.7435, -3.749) (-8.7206, -3.7434) (-8.6979, -3.7374) (-8.6754, -3.7308) (-8.6577, -3.7247) (-8.6447, -3.7197) (-8.636, -3.7161) (-8.6317, -3.7143) knots -1 -1 -1 -1 -1 -1 -0.98571429 -0.97142857 -0.95714286 -0.94285714 -0.92857143 -0.91428571 -0.9 -0.88571429 -0.87142857 -0.85714286 -0.84285714 -0.82857143 -0.81428571 -0.8 -0.78571429 -0.77142857 -0.75714286 -0.74285714 -0.72857143 -0.71428571 -0.7 -0.68571429 -0.67142857 -0.65714286 -0.64285714 -0.62857143 -0.61428571 -0.6 -0.58571429 -0.57142857 -0.55714286 -0.54285714 -0.52857143 -0.51428571 -0.5 -0.48571429 -0.47142857 -0.45714286 -0.44285714 -0.42857143 -0.41428571 -0.4 -0.38571429 -0.37142857 -0.35714286 -0.34285714 -0.32857143 -0.31428571 -0.3 -0.28571429 -0.27142857 -0.25714286 -0.24285714 -0.22857143 -0.21428571 -0.2 -0.18571429 -0.17142857 -0.15714286 -0.14285714 -0.12857143 -0.11428571 -0.1 -0.08571429 -0.07142857 -0.05714286 -0.04285714 -0.02857143 -0.01428571 0 0 0 0 0 0
  line L3 (-8.6317, -3.7143) -> (-8.3939, -3.6119)
  arc A7 (-8.0038, -3.76) -> (-8.3939, -3.6119) centre (-8.2754, -3.8875) ccw
  arc A8 (-8.0038, -3.76) -> (-7.7464, -4.2652) centre (0, 0) ccw
  arc A9 (-7.856, -4.6678) -> (-7.7464, -4.2652) centre (-8.0092, -4.4099) ccw
  line L4 (-7.856, -4.6678) -> (-8.0785, -4.8)
  spline S4 degree 5 poles (-8.0785, -4.8) (-8.0825, -4.8024) (-8.0905, -4.8073) (-8.1023, -4.8149) (-8.1175, -4.8257) (-8.1361, -4.84) (-8.1543, -4.8548) (-8.1723, -4.87) (-8.1901, -4.8854) (-8.2079, -4.901) (-8.2256, -4.9167) (-8.2431, -4.9326) (-8.2605, -4.9487) (-8.2777, -4.9651) (-8.2947, -4.9818) (-8.3116, -4.9987) (-8.3283, -5.0159) (-8.3448, -5.0332) (-8.3612, -5.0507) (-8.3776, -5.0684) (-8.3938, -5.0862) (-8.4099, -5.1042) (-8.4258, -5.1224) (-8.4417, -5.1407) (-8.4574, -5.1592) (-8.473, -5.1778) (-8.4885, -5.1966) (-8.5039, -5.2156) (-8.5192, -5.2347) (-8.5343, -5.2539) (-8.5494, -5.2733) (-8.5643, -5.2928) (-8.5792, -5.3125) (-8.5939, -5.3323) (-8.6085, -5.3522) (-8.6231, -5.3722) (-8.6375, -5.3924) (-8.6518, -5.4127) (-8.666, -5.4331) (-8.6801, -5.4537) (-8.6941, -5.4744) (-8.708, -5.4952) (-8.7218, -5.5161) (-8.7356, -5.5371) (-8.7492, -5.5583) (-8.7627, -5.5795) (-8.7761, -5.6009) (-8.7894, -5.6224) (-8.8026, -5.644) (-8.8158, -5.6657) (-8.8288, -5.6875) (-8.8417, -5.7094) (-8.8545, -5.7314) (-8.8673, -5.7536) (-8.8799, -5.7758) (-8.8925, -5.7981) (-8.9049, -5.8206) (-8.9173, -5.8431) (-8.9295, -5.8657) (-8.9417, -5.8885) (-8.9538, -5.9113) (-8.9657, -5.9343) (-8.9776, -5.9573) (-8.9894, -5.9804) (-9.0011, -6.0036) (-9.0127, -6.0269) (-9.0242, -6.0504) (-9.0356, -6.0739) (-9.0469, -6.0974) (-9.0581, -6.1211) (-9.0692, -6.1449) (-9.0781, -6.164) (-9.0847, -6.1784) (-9.089, -6.1879) (-9.0912, -6.1927) knots 0 0 0 0 0 0 0.01428571 0.02857143 0.04285714 0.05714286 0.07142857 0.08571429 0.1 0.11428571 0.12857143 0.14285714 0.15714286 0.17142857 0.18571429 0.2 0.21428571 0.22857143 0.24285714 0.25714286 0.27142857 0.28571429 0.3 0.31428571 0.32857143 0.34285714 0.35714286 0.37142857 0.38571429 0.4 0.41428571 0.42857143 0.44285714 0.45714286 0.47142857 0.48571429 0.5 0.51428571 0.52857143 0.54285714 0.55714286 0.57142857 0.58571429 0.6 0.61428571 0.62857143 0.64285714 0.65714286 0.67142857 0.68571429 0.7 0.71428571 0.72857143 0.74285714 0.75714286 0.77142857 0.78571429 0.8 0.81428571 0.82857143 0.84285714 0.85714286 0.87142857 0.88571429 0.9 0.91428571 0.92857143 0.94285714 0.95714286 0.97142857 0.98571429 1 1 1 1 1 1
  arc A10 (-9.0912, -6.1927) -> (-8.699, -6.7326) centre (0, 0) ccw
  spline S5 degree 5 poles (-8.699, -6.7326) (-8.6937, -6.732) (-8.6833, -6.7308) (-8.6676, -6.729) (-8.6467, -6.7265) (-8.6207, -6.7233) (-8.5947, -6.7199) (-8.5687, -6.7164) (-8.5429, -6.7128) (-8.517, -6.7091) (-8.4913, -6.7053) (-8.4656, -6.7014) (-8.4399, -6.6973) (-8.4144, -6.6931) (-8.3889, -6.6888) (-8.3634, -6.6844) (-8.338, -6.6799) (-8.3127, -6.6752) (-8.2875, -6.6704) (-8.2623, -6.6655) (-8.2371, -6.6605) (-8.2121, -6.6553) (-8.1871, -6.6501) (-8.1622, -6.6447) (-8.1374, -6.6391) (-8.1126, -6.6335) (-8.0879, -6.6277) (-8.0633, -6.6218) (-8.0387, -6.6158) (-8.0143, -6.6096) (-7.9899, -6.6034) (-7.9655, -6.5969) (-7.9413, -6.5904) (-7.9171, -6.5837) (-7.8931, -6.5769) (-7.8691, -6.57) (-7.8452, -6.5629) (-7.8213, -6.5557) (-7.7976, -6.5484) (-7.774, -6.5409) (-7.7504, -6.5333) (-7.7269, -6.5255) (-7.7036, -6.5176) (-7.6803, -6.5096) (-7.6571, -6.5014) (-7.634, -6.4931) (-7.6111, -6.4846) (-7.5882, -6.476) (-7.5654, -6.4672) (-7.5427, -6.4583) (-7.5202, -6.4492) (-7.4977, -6.44) (-7.4754, -6.4306) (-7.4532, -6.421) (-7.4311, -6.4112) (-7.4092, -6.4013) (-7.3873, -6.3912) (-7.3656, -6.381) (-7.344, -6.3706) (-7.3225, -6.3601) (-7.3012, -6.3493) (-7.28, -6.3383) (-7.2591, -6.327) (-7.2384, -6.3154) (-7.2179, -6.3036) (-7.1975, -6.2917) (-7.1772, -6.2796) (-7.157, -6.2674) (-7.137, -6.255) (-7.1173, -6.2423) (-7.098, -6.229) (-7.083, -6.2178) (-7.0721, -6.209) (-7.065, -6.2029) (-7.0615, -6.1998) knots -1 -1 -1 -1 -1 -1 -0.98571429 -0.97142857 -0.95714286 -0.94285714 -0.92857143 -0.91428571 -0.9 -0.88571429 -0.87142857 -0.85714286 -0.84285714 -0.82857143 -0.81428571 -0.8 -0.78571429 -0.77142857 -0.75714286 -0.74285714 -0.72857143 -0.71428571 -0.7 -0.68571429 -0.67142857 -0.65714286 -0.64285714 -0.62857143 -0.61428571 -0.6 -0.58571429 -0.57142857 -0.55714286 -0.54285714 -0.52857143 -0.51428571 -0.5 -0.48571429 -0.47142857 -0.45714286 -0.44285714 -0.42857143 -0.41428571 -0.4 -0.38571429 -0.37142857 -0.35714286 -0.34285714 -0.32857143 -0.31428571 -0.3 -0.28571429 -0.27142857 -0.25714286 -0.24285714 -0.22857143 -0.21428571 -0.2 -0.18571429 -0.17142857 -0.15714286 -0.14285714 -0.12857143 -0.11428571 -0.1 -0.08571429 -0.07142857 -0.05714286 -0.04285714 -0.02857143 -0.01428571 0 0 0 0 0 0
  line L5 (-7.0615, -6.1998) -> (-6.867, -6.029)
  arc A11 (-6.4502, -6.0492) -> (-6.867, -6.029) centre (-6.669, -6.2545) ccw
  arc A12 (-6.4502, -6.0492) -> (-6.0492, -6.4502) centre (0, 0) ccw
  arc A13 (-6.029, -6.867) -> (-6.0492, -6.4502) centre (-6.2545, -6.669) ccw
  line L6 (-6.029, -6.867) -> (-6.1998, -7.0615)
  spline S6 degree 5 poles (-6.1998, -7.0615) (-6.2029, -7.065) (-6.209, -7.0721) (-6.2178, -7.083) (-6.229, -7.098) (-6.2423, -7.1173) (-6.255, -7.137) (-6.2674, -7.157) (-6.2796, -7.1772) (-6.2917, -7.1975) (-6.3036, -7.2179) (-6.3154, -7.2384) (-6.327, -7.2591) (-6.3383, -7.28) (-6.3493, -7.3012) (-6.3601, -7.3225) (-6.3706, -7.344) (-6.381, -7.3656) (-6.3912, -7.3873) (-6.4013, -7.4092) (-6.4112, -7.4311) (-6.421, -7.4532) (-6.4306, -7.4754) (-6.44, -7.4977) (-6.4492, -7.5202) (-6.4583, -7.5427) (-6.4672, -7.5654) (-6.476, -7.5882) (-6.4846, -7.6111) (-6.4931, -7.634) (-6.5014, -7.6571) (-6.5096, -7.6803) (-6.5176, -7.7036) (-6.5255, -7.7269) (-6.5333, -7.7504) (-6.5409, -7.774) (-6.5484, -7.7976) (-6.5557, -7.8213) (-6.5629, -7.8452) (-6.57, -7.8691) (-6.5769, -7.8931) (-6.5837, -7.9171) (-6.5904, -7.9413) (-6.5969, -7.9655) (-6.6034, -7.9899) (-6.6096, -8.0143) (-6.6158, -8.0387) (-6.6218, -8.0633) (-6.6277, -8.0879) (-6.6335, -8.1126) (-6.6391, -8.1374) (-6.6447, -8.1622) (-6.6501, -8.1871) (-6.6553, -8.2121) (-6.6605, -8.2371) (-6.6655, -8.2623) (-6.6704, -8.2875) (-6.6752, -8.3127) (-6.6799, -8.338) (-6.6844, -8.3634) (-6.6888, -8.3889) (-6.6931, -8.4144) (-6.6973, -8.4399) (-6.7014, -8.4656) (-6.7053, -8.4913) (-6.7091, -8.517) (-6.7128, -8.5429) (-6.7164, -8.5687) (-6.7199, -8.5947) (-6.7233, -8.6207) (-6.7265, -8.6467) (-6.729, -8.6676) (-6.7308, -8.6833) (-6.732, -8.6937) (-6.7326, -8.699) knots 0 0 0 0 0 0 0.01428571 0.02857143 0.04285714 0.05714286 0.07142857 0.08571429 0.1 0.11428571 0.12857143 0.14285714 0.15714286 0.17142857 0.18571429 0.2 0.21428571 0.22857143 0.24285714 0.25714286 0.27142857 0.28571429 0.3 0.31428571 0.32857143 0.34285714 0.35714286 0.37142857 0.38571429 0.4 0.41428571 0.42857143 0.44285714 0.45714286 0.47142857 0.48571429 0.5 0.51428571 0.52857143 0.54285714 0.55714286 0.57142857 0.58571429 0.6 0.61428571 0.62857143 0.64285714 0.65714286 0.67142857 0.68571429 0.7 0.71428571 0.72857143 0.74285714 0.75714286 0.77142857 0.78571429 0.8 0.81428571 0.82857143 0.84285714 0.85714286 0.87142857 0.88571429 0.9 0.91428571 0.92857143 0.94285714 0.95714286 0.97142857 0.98571429 1 1 1 1 1 1
  arc A14 (-6.7326, -8.699) -> (-6.1927, -9.0912) centre (0, 0) ccw